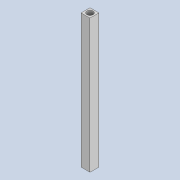
# Autodesk Inventor part: carbon_fiber_150
Saved by Autodesk Inventor 2020 (Build 240168000, 168)
## iProperties
Created: 2022-02-03
Part Number: carbon_fiber_150
Material: Generic
Document SubType Name: Modeling
Designer: Shuang Peng
Density: 1 g/cm^3
Appearance: Default
Author: Shuang Peng
Autodesk Inventor part; units mm, degrees
ref_plane "YZ Plane" through (0, 0, 0) normal (1, 0, 0) x (0, 1, 0)
ref_plane "XZ Plane" through (0, 0, 0) normal (0, 1, 0) x (-1, 0, 0)
ref_plane "XY Plane" through (0, 0, 0) normal (0, 0, 1) x (1, 0, 0)
sketch "Sketch1" plane through (0, 0, 0) normal (0, 1, 0) x (-1, 0, 0)
  line L0 (5, 5) -> (5, -5)
  line L1 (5, -5) -> (-5, -5)
  line L2 (-5, -5) -> (-5, 5)
  line L3 (-5, 5) -> (5, 5)
  line L4 (5, 5) -> (-5, -5) construction
  line L5 (5, -5) -> (-5, 5) construction
  circle A0 centre (0, 0) radius 3.5
  dimension "d0" = 10
  dimension "d1" = 10
  dimension "d2" = 7
  constraints: 12 end point, 2 midpoint, 2 parallel, 1 centre point, 1 coincident, 1 perpendicular, 1 vertical
  measures "d0" distance of L0.start L0.end
  measures "d1" distance of L0.end L1.end
  measures "d2" diameter of A0
extrude "Extrusion1" add sketch "Sketch1" along normal blind 150
body "Solid1"
